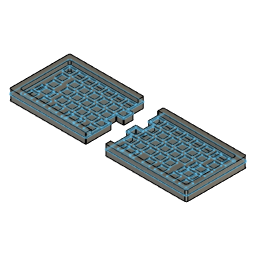
base30_30 (Autodesk Fusion 360 design; units mm, degrees)
Autodesk Fusion 360 part; units mm, degrees
(part 1 of 2)
sketch "kbplate" plane through (0, 0, 0) normal (0, 0, 1) x (1, 0, 0)
  line L0 (231.125, -3.025) -> (231.125, -16.025)
  arc A0 (320.238, -3.025) -> (319.738, -2.525) centre (319.738, -3.025) ccw
  arc A1 (250.175, -16.025) -> (250.675, -16.525) centre (250.675, -16.025) ccw
  line L1 (231.625, -16.525) -> (244.625, -16.525)
  arc A2 (197, -35.575) -> (197.5, -35.075) centre (197, -35.075) ccw
  line L2 (313.738, -17.525) -> (319.738, -17.525)
  line L3 (173.975, -3.025) -> (173.975, -16.025)
  arc A3 (193.025, -16.025) -> (193.525, -16.525) centre (193.525, -16.025) ccw
  arc A4 (212.075, -16.025) -> (212.575, -16.525) centre (212.575, -16.025) ccw
  arc A5 (207.025, -3.025) -> (206.525, -2.525) centre (206.525, -3.025) ccw
  line L4 (250.175, -3.025) -> (250.175, -16.025)
  line L5 (212.575, -16.525) -> (225.575, -16.525)
  line L6 (313.238, -3.025) -> (313.238, -17.025)
  arc A6 (44.6, -35.575) -> (45.1, -35.075) centre (44.6, -35.075) ccw
  arc A7 (297.8, -16.025) -> (298.3, -16.525) centre (298.3, -16.025) ccw
  line L7 (311.8, -16.025) -> (311.8, -3.025)
  arc A8 (250.675, -2.525) -> (250.175, -3.025) centre (250.675, -3.025) ccw
  line L8 (64.15, -35.075) -> (64.15, -22.075)
  arc A9 (197.5, -22.075) -> (197, -21.575) centre (197, -22.075) ccw
  arc A10 (212.575, -2.525) -> (212.075, -3.025) centre (212.575, -3.025) ccw
  line L9 (69.7, -35.575) -> (82.7, -35.575)
  arc A11 (31.1, -35.075) -> (31.6, -35.575) centre (31.6, -35.075) ccw
  arc A12 (183.5, -35.075) -> (184, -35.575) centre (184, -35.075) ccw
  line L10 (320.238, -17.025) -> (320.238, -3.025)
  arc A13 (64.15, -22.075) -> (63.65, -21.575) centre (63.65, -22.075) ccw
  arc A14 (121.3, -22.075) -> (120.8, -21.575) centre (120.8, -22.075) ccw
  line L11 (45.1, -35.075) -> (45.1, -22.075)
  arc A15 (184, -21.575) -> (183.5, -22.075) centre (184, -22.075) ccw
  arc A16 (88.75, -21.575) -> (88.25, -22.075) centre (88.75, -22.075) ccw
  arc A17 (50.15, -35.075) -> (50.65, -35.575) centre (50.65, -35.075) ccw
  arc A18 (101.75, -35.575) -> (102.25, -35.075) centre (101.75, -35.075) ccw
  arc A19 (264.175, -3.025) -> (263.675, -2.525) centre (263.675, -3.025) ccw
  line L12 (206.525, -2.525) -> (193.525, -2.525)
  line L13 (212.075, -3.025) -> (212.075, -16.025)
  arc A20 (69.7, -21.575) -> (69.2, -22.075) centre (69.7, -22.075) ccw
  line L14 (121.3, -35.075) -> (121.3, -22.075)
  line L15 (7.7875, -35.575) -> (20.7875, -35.575)
  arc A21 (313.738, -2.525) -> (313.238, -3.025) centre (313.738, -3.025) ccw
  arc A22 (289.362, -17.025) -> (289.862, -17.525) centre (289.862, -17.025) ccw
  line L16 (283.225, -16.025) -> (283.225, -3.025)
  line L17 (269.225, -3.025) -> (269.225, -16.025)
  line L18 (225.575, -2.525) -> (212.575, -2.525)
  arc A23 (225.575, -16.525) -> (226.075, -16.025) centre (225.575, -16.025) ccw
  arc A24 (226.075, -3.025) -> (225.575, -2.525) centre (225.575, -3.025) ccw
  line L19 (250.675, -16.525) -> (263.675, -16.525)
  arc A25 (263.675, -16.525) -> (264.175, -16.025) centre (263.675, -16.025) ccw
  line L20 (193.025, -3.025) -> (193.025, -16.025)
  line L21 (107.8, -35.575) -> (120.8, -35.575)
  line L22 (120.8, -21.575) -> (107.8, -21.575)
  arc A26 (245.125, -3.025) -> (244.625, -2.525) centre (244.625, -3.025) ccw
  arc A27 (69.2, -35.075) -> (69.7, -35.575) centre (69.7, -35.075) ccw
  line L23 (88.75, -35.575) -> (101.75, -35.575)
  line L24 (184, -35.575) -> (197, -35.575)
  arc A28 (193.525, -2.525) -> (193.025, -3.025) centre (193.525, -3.025) ccw
  arc A29 (21.2875, -22.075) -> (20.7875, -21.575) centre (20.7875, -22.075) ccw
  arc A30 (50.65, -21.575) -> (50.15, -22.075) centre (50.65, -22.075) ccw
  arc A31 (45.1, -22.075) -> (44.6, -21.575) centre (44.6, -22.075) ccw
  line L25 (126.35, -22.075) -> (126.35, -35.075)
  arc A32 (296.362, -3.025) -> (295.862, -2.525) centre (295.862, -3.025) ccw
  line L26 (139.85, -21.575) -> (126.85, -21.575)
  line L27 (7.2875, -22.075) -> (7.2875, -35.075)
  arc A33 (107.8, -21.575) -> (107.3, -22.075) centre (107.8, -22.075) ccw
  line L28 (319.738, -2.525) -> (313.738, -2.525)
  arc A34 (283.225, -3.025) -> (282.725, -2.525) centre (282.725, -3.025) ccw
  line L29 (31.1, -22.075) -> (31.1, -35.075)
  line L30 (69.2, -22.075) -> (69.2, -35.075)
  arc A35 (139.85, -35.575) -> (140.35, -35.075) centre (139.85, -35.075) ccw
  line L31 (50.15, -22.075) -> (50.15, -35.075)
  line L32 (63.65, -21.575) -> (50.65, -21.575)
  line L33 (102.25, -35.075) -> (102.25, -22.075)
  line L34 (50.65, -35.575) -> (63.65, -35.575)
  arc A36 (82.7, -35.575) -> (83.2, -35.075) centre (82.7, -35.075) ccw
  line L35 (88.25, -22.075) -> (88.25, -35.075)
  arc A37 (31.6, -21.575) -> (31.1, -22.075) centre (31.6, -22.075) ccw
  line L36 (107.3, -22.075) -> (107.3, -35.075)
  arc A38 (140.35, -22.075) -> (139.85, -21.575) centre (139.85, -22.075) ccw
  line L37 (140.35, -35.075) -> (140.35, -22.075)
  arc A39 (88.25, -35.075) -> (88.75, -35.575) centre (88.75, -35.075) ccw
  arc A40 (126.85, -21.575) -> (126.35, -22.075) centre (126.85, -22.075) ccw
  line L38 (21.2875, -35.075) -> (21.2875, -22.075)
  line L39 (82.7, -21.575) -> (69.7, -21.575)
  line L40 (44.6, -21.575) -> (31.6, -21.575)
  line L41 (101.75, -21.575) -> (88.75, -21.575)
  arc A41 (20.7875, -35.575) -> (21.2875, -35.075) centre (20.7875, -35.075) ccw
  arc A42 (107.3, -35.075) -> (107.8, -35.575) centre (107.8, -35.075) ccw
  arc A43 (102.25, -22.075) -> (101.75, -21.575) centre (101.75, -22.075) ccw
  line L42 (126.85, -35.575) -> (139.85, -35.575)
  line L43 (31.6, -35.575) -> (44.6, -35.575)
  arc A44 (126.35, -35.075) -> (126.85, -35.575) centre (126.85, -35.075) ccw
  arc A45 (7.2875, -35.075) -> (7.7875, -35.575) centre (7.7875, -35.075) ccw
  line L44 (20.7875, -21.575) -> (7.7875, -21.575)
  arc A46 (63.65, -35.575) -> (64.15, -35.075) centre (63.65, -35.075) ccw
  arc A47 (83.2, -22.075) -> (82.7, -21.575) centre (82.7, -22.075) ccw
  line L45 (83.2, -35.075) -> (83.2, -22.075)
  arc A48 (120.8, -35.575) -> (121.3, -35.075) centre (120.8, -35.075) ccw
  arc A49 (7.7875, -21.575) -> (7.2875, -22.075) centre (7.7875, -22.075) ccw
  line L46 (221.6, -22.075) -> (221.6, -35.075)
  line L47 (316.0625, -21.575) -> (303.0625, -21.575)
  arc A50 (202.55, -35.075) -> (203.05, -35.575) centre (203.05, -35.075) ccw
  line L48 (197.5, -35.075) -> (197.5, -22.075)
  line L49 (303.0625, -35.575) -> (316.0625, -35.575)
  arc A51 (292.25, -35.575) -> (292.75, -35.075) centre (292.25, -35.075) ccw
  line L50 (235.6, -35.075) -> (235.6, -22.075)
  line L51 (222.1, -35.575) -> (235.1, -35.575)
  line L52 (10.1687, -54.625) -> (23.1687, -54.625)
  arc A52 (235.1, -35.575) -> (235.6, -35.075) centre (235.1, -35.075) ccw
  arc A53 (9.6687, -54.125) -> (10.1687, -54.625) centre (10.1687, -54.125) ccw
  arc A54 (303.0625, -21.575) -> (302.5625, -22.075) centre (303.0625, -22.075) ccw
  arc A55 (36.3625, -40.625) -> (35.8625, -41.125) centre (36.3625, -41.125) ccw
  arc A56 (222.1, -21.575) -> (221.6, -22.075) centre (222.1, -22.075) ccw
  line L53 (302.5625, -22.075) -> (302.5625, -35.075)
  line L54 (273.7, -35.075) -> (273.7, -22.075)
  line L55 (36.3625, -54.625) -> (49.3625, -54.625)
  line L56 (23.6687, -54.125) -> (23.6687, -41.125)
  line L57 (292.75, -35.075) -> (292.75, -22.075)
  arc A57 (216.05, -35.575) -> (216.55, -35.075) centre (216.05, -35.075) ccw
  arc A58 (302.5625, -35.075) -> (303.0625, -35.575) centre (303.0625, -35.075) ccw
  arc A59 (254.15, -35.575) -> (254.65, -35.075) centre (254.15, -35.075) ccw
  line L58 (23.1687, -40.625) -> (10.1687, -40.625)
  arc A60 (273.2, -35.575) -> (273.7, -35.075) centre (273.2, -35.075) ccw
  line L59 (235.1, -21.575) -> (222.1, -21.575)
  arc A61 (241.15, -21.575) -> (240.65, -22.075) centre (241.15, -22.075) ccw
  line L60 (273.2, -21.575) -> (260.2, -21.575)
  arc A62 (235.6, -22.075) -> (235.1, -21.575) centre (235.1, -22.075) ccw
  line L61 (292.25, -21.575) -> (279.25, -21.575)
  line L62 (216.55, -35.075) -> (216.55, -22.075)
  line L63 (203.05, -35.575) -> (216.05, -35.575)
  line L64 (241.15, -35.575) -> (254.15, -35.575)
  arc A63 (203.05, -21.575) -> (202.55, -22.075) centre (203.05, -22.075) ccw
  line L65 (202.55, -22.075) -> (202.55, -35.075)
  arc A64 (216.55, -22.075) -> (216.05, -21.575) centre (216.05, -22.075) ccw
  arc A65 (316.0625, -35.575) -> (316.5625, -35.075) centre (316.0625, -35.075) ccw
  line L66 (279.25, -35.575) -> (292.25, -35.575)
  arc A66 (260.2, -21.575) -> (259.7, -22.075) centre (260.2, -22.075) ccw
  line L67 (112.0625, -41.125) -> (112.0625, -54.125)
  arc A67 (169.7125, -40.625) -> (169.2125, -41.125) centre (169.7125, -41.125) ccw
  arc A68 (316.5625, -22.075) -> (316.0625, -21.575) centre (316.0625, -22.075) ccw
  arc A69 (10.1687, -40.625) -> (9.6688, -41.125) centre (10.1687, -41.125) ccw
  arc A70 (49.3625, -54.625) -> (49.8625, -54.125) centre (49.3625, -54.125) ccw
  line L68 (183.5, -22.075) -> (183.5, -35.075)
  arc A71 (183.2125, -41.125) -> (182.7125, -40.625) centre (182.7125, -41.125) ccw
  line L69 (182.7125, -40.625) -> (169.7125, -40.625)
  arc A72 (279.25, -21.575) -> (278.75, -22.075) centre (279.25, -22.075) ccw
  arc A73 (202.2625, -41.125) -> (201.7625, -40.625) centre (201.7625, -41.125) ccw
  arc A74 (54.9125, -54.125) -> (55.4125, -54.625) centre (55.4125, -54.125) ccw
  arc A75 (292.75, -22.075) -> (292.25, -21.575) centre (292.25, -22.075) ccw
  arc A76 (278.75, -35.075) -> (279.25, -35.575) centre (279.25, -35.075) ccw
  arc A77 (273.7, -22.075) -> (273.2, -21.575) centre (273.2, -22.075) ccw
  arc A78 (49.8625, -41.125) -> (49.3625, -40.625) centre (49.3625, -41.125) ccw
  arc A79 (23.6687, -41.125) -> (23.1687, -40.625) centre (23.1687, -41.125) ccw
  arc A80 (207.3125, -54.125) -> (207.8125, -54.625) centre (207.8125, -54.125) ccw
  line L70 (197, -21.575) -> (184, -21.575)
  line L71 (9.6687, -41.125) -> (9.6687, -54.125)
  line L72 (316.5625, -35.075) -> (316.5625, -22.075)
  arc A81 (221.6, -35.075) -> (222.1, -35.575) centre (222.1, -35.075) ccw
  arc A82 (254.65, -22.075) -> (254.15, -21.575) centre (254.15, -22.075) ccw
  line L73 (259.7, -22.075) -> (259.7, -35.075)
  arc A83 (23.1687, -54.625) -> (23.6687, -54.125) centre (23.1687, -54.125) ccw
  line L74 (260.2, -35.575) -> (273.2, -35.575)
  line L75 (254.15, -21.575) -> (241.15, -21.575)
  line L76 (254.65, -35.075) -> (254.65, -22.075)
  line L77 (240.65, -22.075) -> (240.65, -35.075)
  line L78 (216.05, -21.575) -> (203.05, -21.575)
  line L79 (278.75, -22.075) -> (278.75, -35.075)
  arc A84 (259.7, -35.075) -> (260.2, -35.575) centre (260.2, -35.075) ccw
  arc A85 (35.8625, -54.125) -> (36.3625, -54.625) centre (36.3625, -54.125) ccw
  arc A86 (240.65, -35.075) -> (241.15, -35.575) centre (241.15, -35.075) ccw
  line L80 (112.5625, -54.625) -> (125.5625, -54.625)
  arc A87 (188.7625, -40.625) -> (188.2625, -41.125) centre (188.7625, -41.125) ccw
  arc A88 (226.8625, -40.625) -> (226.3625, -41.125) centre (226.8625, -41.125) ccw
  line L81 (183.2125, -54.125) -> (183.2125, -41.125)
  line L82 (226.8625, -54.625) -> (239.8625, -54.625)
  arc A89 (201.7625, -54.625) -> (202.2625, -54.125) centre (201.7625, -54.125) ccw
  arc A90 (182.7125, -54.625) -> (183.2125, -54.125) centre (182.7125, -54.125) ccw
  line L83 (73.9625, -41.125) -> (73.9625, -54.125)
  line L84 (68.9125, -54.125) -> (68.9125, -41.125)
  line L85 (188.7625, -54.625) -> (201.7625, -54.625)
  line L86 (55.4125, -54.625) -> (68.4125, -54.625)
  line L87 (93.5125, -54.625) -> (106.5125, -54.625)
  line L88 (126.0625, -54.125) -> (126.0625, -41.125)
  arc A91 (239.8625, -54.625) -> (240.3625, -54.125) centre (239.8625, -54.125) ccw
  arc A92 (169.2125, -54.125) -> (169.7125, -54.625) centre (169.7125, -54.125) ccw
  line L89 (35.8625, -41.125) -> (35.8625, -54.125)
  line L90 (220.8125, -40.625) -> (207.8125, -40.625)
  arc A93 (112.0625, -54.125) -> (112.5625, -54.625) centre (112.5625, -54.125) ccw
  arc A94 (68.4125, -54.625) -> (68.9125, -54.125) centre (68.4125, -54.125) ccw
  line L91 (107.0125, -54.125) -> (107.0125, -41.125)
  arc A95 (125.5625, -54.625) -> (126.0625, -54.125) centre (125.5625, -54.125) ccw
  arc A96 (74.4625, -40.625) -> (73.9625, -41.125) centre (74.4625, -41.125) ccw
  line L92 (202.2625, -54.125) -> (202.2625, -41.125)
  line L93 (49.3625, -40.625) -> (36.3625, -40.625)
  arc A97 (220.8125, -54.625) -> (221.3125, -54.125) centre (220.8125, -54.125) ccw
  arc A98 (14.4313, -73.175) -> (14.9313, -73.675) centre (14.9313, -73.175) ccw
  line L94 (14.4313, -60.175) -> (14.4313, -73.175)
  arc A99 (12.4932, -74.675) -> (12.9932, -74.175) centre (12.4932, -74.175) ccw
  arc A100 (112.5625, -40.625) -> (112.0625, -41.125) centre (112.5625, -41.125) ccw
  line L95 (125.5625, -40.625) -> (112.5625, -40.625)
  arc A101 (107.0125, -41.125) -> (106.5125, -40.625) centre (106.5125, -41.125) ccw
  line L96 (74.4625, -54.625) -> (87.4625, -54.625)
  arc A102 (93.5125, -40.625) -> (93.0125, -41.125) centre (93.5125, -41.125) ccw
  arc A103 (87.4625, -54.625) -> (87.9625, -54.125) centre (87.4625, -54.125) ccw
  arc A104 (126.0625, -41.125) -> (125.5625, -40.625) centre (125.5625, -41.125) ccw
  line L97 (87.9625, -54.125) -> (87.9625, -41.125)
  arc A105 (73.9625, -54.125) -> (74.4625, -54.625) centre (74.4625, -54.125) ccw
  line L98 (87.4625, -40.625) -> (74.4625, -40.625)
  line L99 (54.9125, -41.125) -> (54.9125, -54.125)
  line L100 (221.3125, -54.125) -> (221.3125, -41.125)
  arc A106 (106.5125, -54.625) -> (107.0125, -54.125) centre (106.5125, -54.125) ccw
  arc A107 (93.0125, -54.125) -> (93.5125, -54.625) centre (93.5125, -54.125) ccw
  arc A108 (240.3625, -41.125) -> (239.8625, -40.625) centre (239.8625, -41.125) ccw
  arc A109 (68.9125, -41.125) -> (68.4125, -40.625) centre (68.4125, -41.125) ccw
  line L101 (106.5125, -40.625) -> (93.5125, -40.625)
  line L102 (68.4125, -40.625) -> (55.4125, -40.625)
  arc A110 (55.4125, -40.625) -> (54.9125, -41.125) centre (55.4125, -41.125) ccw
  line L103 (93.0125, -41.125) -> (93.0125, -54.125)
  line L104 (169.2125, -41.125) -> (169.2125, -54.125)
  line L105 (49.8625, -54.125) -> (49.8625, -41.125)
  arc A111 (188.2625, -54.125) -> (188.7625, -54.625) centre (188.7625, -54.125) ccw
  arc A112 (226.3625, -54.125) -> (226.8625, -54.625) centre (226.8625, -54.125) ccw
  arc A113 (207.8125, -40.625) -> (207.3125, -41.125) centre (207.8125, -41.125) ccw
  line L106 (188.2625, -41.125) -> (188.2625, -54.125)
  arc A114 (87.9625, -41.125) -> (87.4625, -40.625) centre (87.4625, -41.125) ccw
  line L107 (207.3125, -41.125) -> (207.3125, -54.125)
  line L108 (201.7625, -40.625) -> (188.7625, -40.625)
  line L109 (169.7125, -54.625) -> (182.7125, -54.625)
  arc A115 (221.3125, -41.125) -> (220.8125, -40.625) centre (220.8125, -41.125) ccw
  line L110 (207.8125, -54.625) -> (220.8125, -54.625)
  line L111 (278.4625, -54.125) -> (278.4625, -41.125)
  line L112 (245.4125, -41.125) -> (245.4125, -54.125)
  arc A116 (259.4125, -41.125) -> (258.9125, -40.625) centre (258.9125, -41.125) ccw
  line L113 (317.3568, -40.625) -> (311.3568, -40.625)
  arc A117 (311.3567, -40.625) -> (310.8567, -41.125) centre (311.3567, -41.125) ccw
  arc A118 (28.4312, -60.175) -> (27.9312, -59.675) centre (27.9312, -60.175) ccw
  arc A119 (245.4125, -54.125) -> (245.9125, -54.625) centre (245.9125, -54.125) ccw
  arc A120 (309.4187, -41.125) -> (308.9187, -40.625) centre (308.9187, -41.125) ccw
  arc A121 (36.3693, -74.675) -> (36.8693, -74.175) centre (36.3693, -74.175) ccw
  line L114 (317.8567, -55.125) -> (317.8567, -41.125)
  line L115 (5.9932, -60.175) -> (5.9932, -74.175)
  line L116 (309.4187, -54.125) -> (309.4187, -41.125)
  line L117 (293.9808, -55.125) -> (293.9808, -41.125)
  line L118 (258.9125, -40.625) -> (245.9125, -40.625)
  arc A122 (14.9313, -59.675) -> (14.4313, -60.175) centre (14.9313, -60.175) ccw
  arc A123 (293.9808, -41.125) -> (293.4808, -40.625) centre (293.4808, -41.125) ccw
  line L119 (239.8625, -40.625) -> (226.8625, -40.625)
  arc A124 (258.9125, -54.625) -> (259.4125, -54.125) centre (258.9125, -54.125) ccw
  arc A125 (317.8568, -41.125) -> (317.3568, -40.625) centre (317.3568, -41.125) ccw
  arc A126 (6.4933, -59.675) -> (5.9933, -60.175) centre (6.4933, -60.175) ccw
  arc A127 (264.9625, -40.625) -> (264.4625, -41.125) centre (264.9625, -41.125) ccw
  line L120 (28.4313, -73.175) -> (28.4312, -60.175)
  arc A128 (278.4625, -41.125) -> (277.9625, -40.625) centre (277.9625, -41.125) ccw
  arc A129 (317.3568, -55.625) -> (317.8568, -55.125) centre (317.3568, -55.125) ccw
  line L121 (310.8567, -41.125) -> (310.8567, -55.125)
  arc A130 (295.9188, -40.625) -> (295.4188, -41.125) centre (295.9188, -41.125) ccw
  arc A131 (245.9125, -40.625) -> (245.4125, -41.125) centre (245.9125, -41.125) ccw
  arc A132 (295.4188, -54.125) -> (295.9188, -54.625) centre (295.9188, -54.125) ccw
  line L122 (240.3625, -54.125) -> (240.3625, -41.125)
  arc A133 (286.9808, -55.125) -> (287.4808, -55.625) centre (287.4808, -55.125) ccw
  line L123 (27.9312, -59.675) -> (14.9313, -59.675)
  arc A134 (29.8693, -74.175) -> (30.3693, -74.675) centre (30.3693, -74.175) ccw
  line L124 (6.4933, -74.675) -> (12.4932, -74.675)
  arc A135 (27.9312, -73.675) -> (28.4312, -73.175) centre (27.9312, -73.175) ccw
  line L125 (14.9313, -73.675) -> (27.9312, -73.675)
  line L126 (259.4125, -54.125) -> (259.4125, -41.125)
  line L127 (245.9125, -54.625) -> (258.9125, -54.625)
  arc A136 (293.4808, -55.625) -> (293.9808, -55.125) centre (293.4808, -55.125) ccw
  line L128 (36.8693, -74.175) -> (36.8693, -60.175)
  line L129 (211.2875, -59.675) -> (198.2875, -59.675)
  line L130 (12.9932, -74.175) -> (12.9932, -60.175)
  line L131 (311.3567, -55.625) -> (317.3567, -55.625)
  line L132 (192.7375, -73.175) -> (192.7375, -60.175)
  line L133 (12.4932, -59.675) -> (6.4932, -59.675)
  line L134 (308.9187, -40.625) -> (295.9188, -40.625)
  line L135 (293.4808, -40.625) -> (287.4808, -40.625)
  arc A137 (12.9932, -60.175) -> (12.4932, -59.675) centre (12.4932, -60.175) ccw
  arc A138 (36.8693, -60.175) -> (36.3693, -59.675) centre (36.3693, -60.175) ccw
  arc A139 (264.4625, -54.125) -> (264.9625, -54.625) centre (264.9625, -54.125) ccw
  line L136 (295.4187, -41.125) -> (295.4187, -54.125)
  line L137 (295.9188, -54.625) -> (308.9188, -54.625)
  line L138 (287.4808, -55.625) -> (293.4808, -55.625)
  line L139 (286.9808, -41.125) -> (286.9808, -55.125)
  arc A140 (277.9625, -54.625) -> (278.4625, -54.125) centre (277.9625, -54.125) ccw
  line L140 (264.4625, -41.125) -> (264.4625, -54.125)
  arc A141 (287.4808, -40.625) -> (286.9808, -41.125) centre (287.4808, -41.125) ccw
  arc A142 (5.9932, -74.175) -> (6.4933, -74.675) centre (6.4933, -74.175) ccw
  line L141 (277.9625, -40.625) -> (264.9625, -40.625)
  line L142 (30.3693, -74.675) -> (36.3693, -74.675)
  arc A143 (310.8567, -55.125) -> (311.3567, -55.625) centre (311.3567, -55.125) ccw
  arc A144 (308.9187, -54.625) -> (309.4187, -54.125) centre (308.9187, -54.125) ccw
  line L143 (264.9625, -54.625) -> (277.9625, -54.625)
  arc A145 (30.3693, -59.675) -> (29.8693, -60.175) centre (30.3693, -60.175) ccw
  line L144 (226.3625, -41.125) -> (226.3625, -54.125)
  line L145 (178.7375, -60.175) -> (178.7375, -73.175)
  line L146 (197.7875, -60.175) -> (197.7875, -73.175)
  arc A146 (102.5375, -73.175) -> (103.0375, -73.675) centre (103.0375, -73.175) ccw
  arc A147 (211.7875, -60.175) -> (211.2875, -59.675) centre (211.2875, -60.175) ccw
  line L147 (102.5375, -60.175) -> (102.5375, -73.175)
  arc A148 (217.3375, -59.675) -> (216.8375, -60.175) centre (217.3375, -60.175) ccw
  line L148 (29.8693, -60.175) -> (29.8693, -74.175)
  line L149 (45.3875, -60.175) -> (45.3875, -73.175)
  arc A149 (198.2875, -59.675) -> (197.7875, -60.175) centre (198.2875, -60.175) ccw
  line L150 (116.5375, -73.175) -> (116.5375, -60.175)
  arc A150 (192.2375, -73.675) -> (192.7375, -73.175) centre (192.2375, -73.175) ccw
  line L151 (135.5875, -73.175) -> (135.5875, -60.175)
  line L152 (59.3875, -73.175) -> (59.3875, -60.175)
  arc A151 (121.5875, -73.175) -> (122.0875, -73.675) centre (122.0875, -73.175) ccw
  line L153 (78.4375, -73.175) -> (78.4375, -60.175)
  line L154 (179.2375, -73.675) -> (192.2375, -73.675)
  line L155 (211.7875, -73.175) -> (211.7875, -60.175)
  line L156 (103.0375, -73.675) -> (116.0375, -73.675)
  line L157 (83.4875, -60.175) -> (83.4875, -73.175)
  arc A152 (178.7375, -73.175) -> (179.2375, -73.675) centre (179.2375, -73.175) ccw
  arc A153 (97.4875, -60.175) -> (96.9875, -59.675) centre (96.9875, -60.175) ccw
  line L158 (306.5942, -74.675) -> (312.5942, -74.675)
  line L159 (5.4062, -92.725) -> (18.4063, -92.725)
  line L160 (4.9062, -79.225) -> (4.9062, -92.225)
  arc A154 (116.5375, -60.175) -> (116.0375, -59.675) centre (116.0375, -60.175) ccw
  arc A155 (116.0375, -73.675) -> (116.5375, -73.175) centre (116.0375, -73.175) ccw
  arc A156 (64.9375, -59.675) -> (64.4375, -60.175) centre (64.9375, -60.175) ccw
  arc A157 (135.5875, -60.175) -> (135.0875, -59.675) centre (135.0875, -60.175) ccw
  line L161 (45.8875, -73.675) -> (58.8875, -73.675)
  arc A158 (45.8875, -59.675) -> (45.3875, -60.175) centre (45.8875, -60.175) ccw
  line L162 (96.9875, -59.675) -> (83.9875, -59.675)
  arc A159 (64.4375, -73.175) -> (64.9375, -73.675) centre (64.9375, -73.175) ccw
  line L163 (77.9375, -59.675) -> (64.9375, -59.675)
  line L164 (116.0375, -59.675) -> (103.0375, -59.675)
  arc A160 (135.0875, -73.675) -> (135.5875, -73.175) centre (135.0875, -73.175) ccw
  line L165 (83.9875, -73.675) -> (96.9875, -73.675)
  arc A161 (192.7375, -60.175) -> (192.2375, -59.675) centre (192.2375, -60.175) ccw
  arc A162 (230.8375, -60.175) -> (230.3375, -59.675) centre (230.3375, -60.175) ccw
  line L166 (198.2875, -73.675) -> (211.2875, -73.675)
  line L167 (97.4875, -73.175) -> (97.4875, -60.175)
  arc A163 (59.3875, -60.175) -> (58.8875, -59.675) centre (58.8875, -60.175) ccw
  arc A164 (77.9375, -73.675) -> (78.4375, -73.175) centre (77.9375, -73.175) ccw
  arc A165 (83.9875, -59.675) -> (83.4875, -60.175) centre (83.9875, -60.175) ccw
  arc A166 (103.0375, -59.675) -> (102.5375, -60.175) centre (103.0375, -60.175) ccw
  arc A167 (122.0875, -59.675) -> (121.5875, -60.175) centre (122.0875, -60.175) ccw
  line L168 (192.2375, -59.675) -> (179.2375, -59.675)
  arc A168 (211.2875, -73.675) -> (211.7875, -73.175) centre (211.2875, -73.175) ccw
  line L169 (64.4375, -60.175) -> (64.4375, -73.175)
  line L170 (122.0875, -73.675) -> (135.0875, -73.675)
  arc A169 (179.2375, -59.675) -> (178.7375, -60.175) centre (179.2375, -60.175) ccw
  arc A170 (78.4375, -60.175) -> (77.9375, -59.675) centre (77.9375, -60.175) ccw
  arc A171 (197.7875, -73.175) -> (198.2875, -73.675) centre (198.2875, -73.175) ccw
  line L171 (217.3375, -73.675) -> (230.3375, -73.675)
  arc A172 (83.4875, -73.175) -> (83.9875, -73.675) centre (83.9875, -73.175) ccw
  line L172 (135.0875, -59.675) -> (122.0875, -59.675)
  line L173 (64.9375, -73.675) -> (77.9375, -73.675)
  line L174 (58.8875, -59.675) -> (45.8875, -59.675)
  arc A173 (216.8375, -73.175) -> (217.3375, -73.675) centre (217.3375, -73.175) ccw
  arc A174 (45.3875, -73.175) -> (45.8875, -73.675) centre (45.8875, -73.175) ccw
  arc A175 (96.9875, -73.675) -> (97.4875, -73.175) centre (96.9875, -73.175) ccw
  line L175 (121.5875, -60.175) -> (121.5875, -73.175)
  arc A176 (58.8875, -73.675) -> (59.3875, -73.175) centre (58.8875, -73.175) ccw
  arc A177 (230.3375, -73.675) -> (230.8375, -73.175) centre (230.3375, -73.175) ccw
  line L176 (36.3693, -59.675) -> (30.3693, -59.675)
  line L177 (312.5942, -59.675) -> (306.5942, -59.675)
  line L178 (304.6562, -73.175) -> (304.6562, -60.175)
  line L179 (254.9375, -60.175) -> (254.9375, -73.175)
  arc A178 (29.2188, -78.725) -> (28.7188, -79.225) centre (29.2188, -79.225) ccw
  arc A179 (282.7183, -59.675) -> (282.2183, -60.175) centre (282.7183, -60.175) ccw
  line L180 (249.8875, -73.175) -> (249.8875, -60.175)
  line L181 (249.3875, -59.675) -> (236.3875, -59.675)
  line L182 (230.3375, -59.675) -> (217.3375, -59.675)
  arc A180 (288.7183, -74.675) -> (289.2183, -74.175) centre (288.7183, -74.175) ccw
  arc A181 (268.4375, -73.675) -> (268.9375, -73.175) centre (268.4375, -73.175) ccw
  line L183 (282.2183, -60.175) -> (282.2183, -74.175)
  line L184 (291.1562, -73.675) -> (304.1562, -73.675)
  arc A182 (42.7188, -79.225) -> (42.2188, -78.725) centre (42.2188, -79.225) ccw
  line L185 (304.1562, -59.675) -> (291.1562, -59.675)
  arc A183 (268.9375, -60.175) -> (268.4375, -59.675) centre (268.4375, -60.175) ccw
  line L186 (216.8375, -60.175) -> (216.8375, -73.175)
  line L187 (282.7183, -74.675) -> (288.7183, -74.675)
  line L188 (313.0942, -74.175) -> (313.0942, -60.175)
  arc A184 (4.9062, -92.225) -> (5.4062, -92.725) centre (5.4062, -92.225) ccw
  line L189 (289.2183, -74.175) -> (289.2183, -60.175)
  line L190 (268.4375, -59.675) -> (255.4375, -59.675)
  arc A185 (289.2183, -60.175) -> (288.7183, -59.675) centre (288.7183, -60.175) ccw
  line L191 (268.9375, -73.175) -> (268.9375, -60.175)
  line L192 (288.7183, -59.675) -> (282.7183, -59.675)
  arc A186 (249.3875, -73.675) -> (249.8875, -73.175) centre (249.3875, -73.175) ccw
  arc A187 (18.9062, -79.225) -> (18.4062, -78.725) centre (18.4062, -79.225) ccw
  arc A188 (18.4062, -92.725) -> (18.9063, -92.225) centre (18.4062, -92.225) ccw
  arc A189 (28.7188, -92.225) -> (29.2188, -92.725) centre (29.2188, -92.225) ccw
  arc A190 (291.1562, -59.675) -> (290.6562, -60.175) centre (291.1562, -60.175) ccw
  line L193 (29.2188, -92.725) -> (42.2188, -92.725)
  line L194 (42.2188, -78.725) -> (29.2188, -78.725)
  arc A191 (306.0942, -74.175) -> (306.5942, -74.675) centre (306.5942, -74.175) ccw
  line L195 (306.0942, -60.175) -> (306.0942, -74.175)
  line L196 (42.7188, -92.225) -> (42.7188, -79.225)
  line L197 (255.4375, -73.675) -> (268.4375, -73.675)
  arc A192 (290.6562, -73.175) -> (291.1562, -73.675) centre (291.1562, -73.175) ccw
  arc A193 (304.1562, -73.675) -> (304.6562, -73.175) centre (304.1562, -73.175) ccw
  arc A194 (282.2183, -74.175) -> (282.7183, -74.675) centre (282.7183, -74.175) ccw
  line L198 (290.6562, -60.175) -> (290.6562, -73.175)
  arc A195 (304.6562, -60.175) -> (304.1562, -59.675) centre (304.1562, -60.175) ccw
  arc A196 (306.5942, -59.675) -> (306.0942, -60.175) centre (306.5942, -60.175) ccw
  arc A197 (249.8875, -60.175) -> (249.3875, -59.675) centre (249.3875, -60.175) ccw
  line L199 (18.4062, -78.725) -> (5.4062, -78.725)
  arc A198 (42.2188, -92.725) -> (42.7188, -92.225) centre (42.2188, -92.225) ccw
  arc A199 (254.9375, -73.175) -> (255.4375, -73.675) centre (255.4375, -73.175) ccw
  arc A200 (66.5312, -79.225) -> (66.0312, -78.725) centre (66.0312, -79.225) ccw
  arc A201 (312.5942, -74.675) -> (313.0942, -74.175) centre (312.5942, -74.175) ccw
  line L200 (236.3875, -73.675) -> (249.3875, -73.675)
  arc A202 (52.5313, -92.225) -> (53.0313, -92.725) centre (53.0313, -92.225) ccw
  arc A203 (313.0942, -60.175) -> (312.5942, -59.675) centre (312.5942, -60.175) ccw
  line L201 (230.8375, -73.175) -> (230.8375, -60.175)
  arc A204 (66.0312, -92.725) -> (66.5312, -92.225) centre (66.0312, -92.225) ccw
  arc A205 (235.8875, -73.175) -> (236.3875, -73.675) centre (236.3875, -73.175) ccw
  arc A206 (255.4375, -59.675) -> (254.9375, -60.175) centre (255.4375, -60.175) ccw
  line L202 (28.7188, -79.225) -> (28.7188, -92.225)
  line L203 (235.8875, -60.175) -> (235.8875, -73.175)
  line L204 (18.9063, -92.225) -> (18.9063, -79.225)
  arc A207 (5.4062, -78.725) -> (4.9063, -79.225) centre (5.4062, -79.225) ccw
  arc A208 (236.3875, -59.675) -> (235.8875, -60.175) centre (236.3875, -60.175) ccw
  arc A209 (83.9308, -93.725) -> (84.4308, -93.225) centre (83.9308, -93.225) ccw
  line L205 (101.8068, -93.725) -> (107.8068, -93.725)
  line L206 (217.3443, -78.725) -> (211.3442, -78.725)
  arc A210 (247.5063, -79.225) -> (247.0063, -78.725) centre (247.0063, -79.225) ccw
  line L207 (66.0312, -78.725) -> (53.0312, -78.725)
  line L208 (86.3688, -92.725) -> (99.3688, -92.725)
  arc A211 (211.3442, -78.725) -> (210.8442, -79.225) centre (211.3442, -79.225) ccw
  line L209 (53.0313, -92.725) -> (66.0312, -92.725)
  line L210 (66.5312, -92.225) -> (66.5312, -79.225)
  arc A212 (77.4308, -93.225) -> (77.9308, -93.725) centre (77.9308, -93.225) ccw
  line L211 (83.9308, -78.725) -> (77.9308, -78.725)
  arc A213 (186.9683, -93.225) -> (187.4683, -93.725) centre (187.4683, -93.225) ccw
  line L212 (195.9063, -92.725) -> (208.9062, -92.725)
  arc A214 (234.0063, -78.725) -> (233.5063, -79.225) centre (234.0063, -79.225) ccw
  line L213 (209.4062, -92.225) -> (209.4062, -79.225)
  line L214 (186.9683, -79.225) -> (186.9683, -93.225)
  line L215 (234.0063, -92.725) -> (247.0063, -92.725)
  arc A215 (133.2063, -79.225) -> (132.7063, -78.725) centre (132.7063, -79.225) ccw
  line L216 (99.8688, -92.225) -> (99.8688, -79.225)
  line L217 (119.7062, -92.725) -> (132.7063, -92.725)
  arc A216 (195.4063, -92.225) -> (195.9063, -92.725) centre (195.9063, -92.225) ccw
  arc A217 (107.8068, -93.725) -> (108.3068, -93.225) centre (107.8068, -93.225) ccw
  line L218 (119.2063, -79.225) -> (119.2063, -92.225)
  arc A218 (247.0063, -92.725) -> (247.5063, -92.225) centre (247.0063, -92.225) ccw
  arc A219 (210.8442, -93.225) -> (211.3442, -93.725) centre (211.3442, -93.225) ccw
  line L219 (217.8442, -93.225) -> (217.8442, -79.225)
  line L220 (84.4308, -93.225) -> (84.4308, -79.225)
  line L221 (187.4683, -93.725) -> (193.4683, -93.725)
  arc A220 (99.8688, -79.225) -> (99.3688, -78.725) centre (99.3688, -79.225) ccw
  arc A221 (119.7062, -78.725) -> (119.2062, -79.225) centre (119.7062, -79.225) ccw
  arc A222 (84.4308, -79.225) -> (83.9308, -78.725) centre (83.9308, -79.225) ccw
  arc A223 (233.5063, -92.225) -> (234.0063, -92.725) centre (234.0063, -92.225) ccw
  line L222 (77.9308, -93.725) -> (83.9308, -93.725)
  arc A224 (101.3067, -93.225) -> (101.8068, -93.725) centre (101.8068, -93.225) ccw
  arc A225 (101.8068, -78.725) -> (101.3068, -79.225) centre (101.8068, -79.225) ccw
  arc A226 (208.9062, -92.725) -> (209.4062, -92.225) centre (208.9062, -92.225) ccw
  line L223 (193.4683, -78.725) -> (187.4683, -78.725)
  line L224 (211.3442, -93.725) -> (217.3442, -93.725)
  line L225 (208.9062, -78.725) -> (195.9063, -78.725)
  arc A227 (132.7063, -92.725) -> (133.2063, -92.225) centre (132.7063, -92.225) ccw
  arc A228 (119.2062, -92.225) -> (119.7062, -92.725) centre (119.7062, -92.225) ccw
  line L226 (193.9683, -93.225) -> (193.9683, -79.225)
  arc A229 (108.3068, -79.225) -> (107.8068, -78.725) centre (107.8068, -79.225) ccw
  line L227 (195.4063, -79.225) -> (195.4063, -92.225)
  line L228 (101.3067, -79.225) -> (101.3067, -93.225)
  line L229 (85.8688, -79.225) -> (85.8688, -92.225)
  line L230 (133.2063, -92.225) -> (133.2063, -79.225)
  line L231 (107.8068, -78.725) -> (101.8068, -78.725)
  line L232 (210.8442, -79.225) -> (210.8442, -93.225)
  arc A230 (193.9683, -79.225) -> (193.4683, -78.725) centre (193.4683, -79.225) ccw
  arc A231 (209.4062, -79.225) -> (208.9062, -78.725) centre (208.9062, -79.225) ccw
  line L233 (99.3688, -78.725) -> (86.3688, -78.725)
  line L234 (108.3068, -93.225) -> (108.3068, -79.225)
  arc A232 (85.8688, -92.225) -> (86.3688, -92.725) centre (86.3688, -92.225) ccw
  arc A233 (53.0313, -78.725) -> (52.5313, -79.225) centre (53.0313, -79.225) ccw
  arc A234 (195.9063, -78.725) -> (195.4063, -79.225) centre (195.9063, -79.225) ccw
  arc A235 (99.3688, -92.725) -> (99.8688, -92.225) centre (99.3688, -92.225) ccw
  arc A236 (77.9308, -78.725) -> (77.4308, -79.225) centre (77.9308, -79.225) ccw
  line L235 (52.5313, -79.225) -> (52.5313, -92.225)
  arc A237 (187.4683, -78.725) -> (186.9683, -79.225) centre (187.4683, -79.225) ccw
  line L236 (132.7063, -78.725) -> (119.7062, -78.725)
  arc A238 (86.3688, -78.725) -> (85.8688, -79.225) centre (86.3688, -79.225) ccw
  arc A239 (217.8443, -79.225) -> (217.3443, -78.725) centre (217.3443, -79.225) ccw
  arc A240 (217.3443, -93.725) -> (217.8443, -93.225) centre (217.3443, -93.225) ccw
  arc A241 (193.4683, -93.725) -> (193.9683, -93.225) centre (193.4683, -93.225) ccw
  line L237 (77.4308, -79.225) -> (77.4308, -93.225)
  line L238 (174.475, -16.525) -> (187.475, -16.525)
  arc A242 (21.575, -16.025) -> (22.075, -16.525) centre (22.075, -16.025) ccw
  line L239 (294.6313, -78.725) -> (281.6313, -78.725)
  line L240 (3.025, -16.525) -> (16.025, -16.525)
  arc A243 (54.625, -3.025) -> (54.125, -2.525) centre (54.125, -3.025) ccw
  line L241 (60.175, -16.525) -> (73.175, -16.525)
  arc A244 (257.3188, -92.225) -> (257.8188, -92.725) centre (257.8188, -92.225) ccw
  arc A245 (304.9438, -92.225) -> (305.4438, -92.725) centre (305.4438, -92.225) ccw
  line L242 (35.075, -2.525) -> (22.075, -2.525)
  arc A246 (73.175, -16.525) -> (73.675, -16.025) centre (73.175, -16.025) ccw
  line L243 (92.225, -2.525) -> (79.225, -2.525)
  line L244 (305.4438, -92.725) -> (318.4438, -92.725)
  line L245 (130.3254, -2.5361) -> (117.325, -2.525)
  arc A247 (22.075, -2.525) -> (21.575, -3.025) centre (22.075, -3.025) ccw
  line L246 (247.5063, -92.225) -> (247.5063, -79.225)
  line L247 (281.1313, -79.225) -> (281.1313, -92.225)
  arc A248 (111.275, -16.525) -> (111.775, -16.025) centre (111.275, -16.025) ccw
  arc A249 (2.525, -16.025) -> (3.025, -16.525) centre (3.025, -16.025) ccw
  arc A250 (271.3188, -79.225) -> (270.8188, -78.725) centre (270.8188, -79.225) ccw
  line L248 (304.9438, -79.225) -> (304.9437, -92.225)
  line L249 (111.275, -2.525) -> (98.275, -2.525)
  arc A251 (294.6313, -92.725) -> (295.1313, -92.225) centre (294.6313, -92.225) ccw
  arc A252 (60.175, -2.525) -> (59.675, -3.025) centre (60.175, -3.025) ccw
  arc A253 (78.725, -16.025) -> (79.225, -16.525) centre (79.225, -16.025) ccw
  line L250 (40.625, -3.025) -> (40.625, -16.025)
  line L251 (92.725, -16.025) -> (92.725, -3.025)
  line L252 (73.175, -2.525) -> (60.175, -2.525)
  line L253 (16.525, -16.025) -> (16.525, -3.025)
  line L254 (281.6313, -92.725) -> (294.6313, -92.725)
  line L255 (111.775, -16.025) -> (111.775, -3.025)
  arc A254 (41.125, -2.525) -> (40.625, -3.025) centre (41.125, -3.025) ccw
  line L256 (21.575, -3.025) -> (21.575, -16.025)
  arc A255 (318.4438, -92.725) -> (318.9438, -92.225) centre (318.4438, -92.225) ccw
  line L257 (233.5063, -79.225) -> (233.5063, -92.225)
  line L258 (270.8188, -78.725) -> (257.8188, -78.725)
  line L259 (318.9438, -92.225) -> (318.9438, -79.225)
  arc A256 (295.1313, -79.225) -> (294.6313, -78.725) centre (294.6313, -79.225) ccw
  arc A257 (16.525, -3.025) -> (16.025, -2.525) centre (16.025, -3.025) ccw
  arc A258 (318.9438, -79.225) -> (318.4438, -78.725) centre (318.4438, -79.225) ccw
  arc A259 (174.475, -2.525) -> (173.975, -3.025) centre (174.475, -3.025) ccw
  line L260 (295.1313, -92.225) -> (295.1313, -79.225)
  arc A260 (35.575, -3.025) -> (35.075, -2.525) centre (35.075, -3.025) ccw
  arc A261 (92.725, -3.025) -> (92.225, -2.525) centre (92.225, -3.025) ccw
  line L261 (257.3188, -79.225) -> (257.3188, -92.225)
  arc A262 (305.4438, -78.725) -> (304.9438, -79.225) centre (305.4438, -79.225) ccw
  line L262 (318.4438, -78.725) -> (305.4438, -78.725)
  arc A263 (116.825, -16.025) -> (117.325, -16.525) centre (117.325, -16.025) ccw
  line L263 (271.3188, -92.225) -> (271.3188, -79.225)
  arc A264 (111.775, -3.025) -> (111.275, -2.525) centre (111.275, -3.025) ccw
  arc A265 (257.8188, -78.725) -> (257.3188, -79.225) centre (257.8188, -79.225) ccw
  line L264 (41.125, -16.525) -> (54.125, -16.525)
  arc A266 (281.1313, -92.225) -> (281.6313, -92.725) centre (281.6313, -92.225) ccw
  arc A267 (40.625, -16.025) -> (41.125, -16.525) centre (41.125, -16.025) ccw
  arc A268 (35.075, -16.525) -> (35.575, -16.025) centre (35.075, -16.025) ccw
  line L265 (247.0063, -78.725) -> (234.0063, -78.725)
  arc A269 (92.225, -16.525) -> (92.725, -16.025) centre (92.225, -16.025) ccw
  line L266 (257.8188, -92.725) -> (270.8188, -92.725)
  arc A270 (54.125, -16.525) -> (54.625, -16.025) centre (54.125, -16.025) ccw
  arc A271 (117.325, -2.525) -> (116.825, -3.025) centre (117.325, -3.025) ccw
  arc A272 (281.6313, -78.725) -> (281.1313, -79.225) centre (281.6313, -79.225) ccw
  line L267 (16.025, -2.525) -> (3.025, -2.525)
  line L268 (35.575, -16.025) -> (35.575, -3.025)
  arc A273 (270.8188, -92.725) -> (271.3188, -92.225) centre (270.8188, -92.225) ccw
  line L269 (117.325, -16.525) -> (130.3253, -16.518)
  line L270 (264.175, -16.025) -> (264.175, -3.025)
  arc A274 (59.675, -16.025) -> (60.175, -16.525) centre (60.175, -16.025) ccw
  line L271 (311.3, -2.525) -> (298.3, -2.525)
  line L272 (289.362, -3.025) -> (289.362, -17.025)
  arc A275 (3.025, -2.525) -> (2.525, -3.025) centre (3.025, -3.025) ccw
  arc A276 (231.125, -16.025) -> (231.625, -16.525) centre (231.625, -16.025) ccw
  line L273 (78.725, -3.025) -> (78.725, -16.025)
  arc A277 (173.975, -16.025) -> (174.475, -16.525) centre (174.475, -16.025) ccw
  arc A278 (206.525, -16.525) -> (207.025, -16.025) centre (206.525, -16.025) ccw
  arc A279 (295.862, -17.525) -> (296.362, -17.025) centre (295.862, -17.025) ccw
  line L274 (269.725, -16.525) -> (282.725, -16.525)
  arc A280 (269.725, -2.525) -> (269.225, -3.025) centre (269.725, -3.025) ccw
  arc A281 (289.862, -2.525) -> (289.362, -3.025) centre (289.862, -3.025) ccw
  line L275 (289.862, -17.525) -> (295.862, -17.525)
  line L276 (297.8, -3.025) -> (297.8, -16.025)
  line L277 (98.275, -16.525) -> (111.275, -16.525)
  line L278 (54.625, -16.025) -> (54.625, -3.025)
  line L279 (187.975, -16.025) -> (187.975, -3.025)
  line L280 (226.075, -16.025) -> (226.075, -3.025)
  line L281 (244.625, -2.525) -> (231.625, -2.525)
  line L282 (97.775, -3.025) -> (97.775, -16.025)
  arc A282 (282.725, -16.525) -> (283.225, -16.025) centre (282.725, -16.025) ccw
  line L283 (2.525, -3.025) -> (2.525, -16.025)
  line L284 (207.025, -16.025) -> (207.025, -3.025)
  line L285 (263.675, -2.525) -> (250.675, -2.525)
  line L286 (296.362, -17.025) -> (296.362, -3.025)
  line L287 (193.525, -16.525) -> (206.525, -16.525)
  line L288 (282.725, -2.525) -> (269.725, -2.525)
  line L289 (298.3, -16.525) -> (311.3, -16.525)
  arc A283 (313.238, -17.025) -> (313.738, -17.525) centre (313.738, -17.025) ccw
  arc A284 (97.775, -16.025) -> (98.275, -16.525) centre (98.275, -16.025) ccw
  arc A285 (187.475, -16.525) -> (187.975, -16.025) centre (187.475, -16.025) ccw
  arc A286 (16.025, -16.525) -> (16.525, -16.025) centre (16.025, -16.025) ccw
  line L290 (59.675, -3.025) -> (59.675, -16.025)
  arc A287 (79.225, -2.525) -> (78.725, -3.025) centre (79.225, -3.025) ccw
  arc A288 (244.625, -16.525) -> (245.125, -16.025) centre (244.625, -16.025) ccw
  arc A289 (319.738, -17.525) -> (320.238, -17.025) centre (319.738, -17.025) ccw
  arc A290 (311.8, -3.025) -> (311.3, -2.525) centre (311.3, -3.025) ccw
  arc A291 (231.625, -2.525) -> (231.125, -3.025) centre (231.625, -3.025) ccw
  line L291 (79.225, -16.525) -> (92.225, -16.525)
  line L292 (73.675, -16.025) -> (73.675, -3.025)
  line L293 (295.862, -2.525) -> (289.862, -2.525)
  arc A292 (98.275, -2.525) -> (97.775, -3.025) centre (98.275, -3.025) ccw
  arc A293 (73.675, -3.025) -> (73.175, -2.525) centre (73.175, -3.025) ccw
  line L294 (245.125, -16.025) -> (245.125, -3.025)
  arc A294 (187.975, -3.025) -> (187.475, -2.525) centre (187.475, -3.025) ccw
  line L295 (116.825, -3.025) -> (116.825, -16.025)
  line L296 (54.125, -2.525) -> (41.125, -2.525)
  arc A295 (311.3, -16.525) -> (311.8, -16.025) centre (311.3, -16.025) ccw
  line L297 (187.475, -2.525) -> (174.475, -2.525)
  line L298 (22.075, -16.525) -> (35.075, -16.525)
  arc A296 (298.3, -2.525) -> (297.8, -3.025) centre (298.3, -3.025) ccw
  arc A297 (269.225, -16.025) -> (269.725, -16.525) centre (269.725, -16.025) ccw
  line L299 (132.35, 0.475) -> (2.525, 0.475)
  line L300 (-0.475, -2.525) -> (-0.475, -93.725)
  line L301 (2.525, -96.725) -> (137.1125, -96.725)
  line L302 (323.238, -93.725) -> (323.238, -2.525)
  line L303 (142.875, -37.1) -> (142.875, -20.05)
  line L304 (141.875, -19.05) -> (134.35, -19.05)
  line L305 (129.5875, -38.1) -> (141.875, -38.1)
  line L306 (128.5875, -56.15) -> (128.5875, -39.1)
  line L307 (137.1125, -57.15) -> (129.5875, -57.15)
  line L308 (138.1125, -105.725) -> (138.1125, -58.15)
  line L309 (177.2125, -96.725) -> (320.238, -96.725)
  line L310 (171.45, 9.475) -> (171.45, -18.05)
  line L311 (320.238, 0.475) -> (172.45, 0.475)
  line L312 (172.45, -19.05) -> (179.975, -19.05)
  line L313 (180.975, -20.05) -> (180.975, -37.1)
  line L314 (179.975, -38.1) -> (167.6875, -38.1)
  line L315 (166.6875, -39.1) -> (166.6875, -56.15)
  line L316 (167.6875, -57.15) -> (175.2125, -57.15)
  line L317 (176.2125, -58.15) -> (176.2125, -105.725)
  arc A298 (2.525, 0.475) -> (-0.475, -2.525) centre (2.525, -2.525) ccw
  arc A299 (-0.475, -93.725) -> (2.525, -96.725) centre (2.525, -93.725) ccw
  arc A300 (137.1125, -96.725) -> (138.1125, -95.725) centre (137.1125, -95.725) ccw
  arc A301 (138.1125, -58.15) -> (137.1125, -57.15) centre (137.1125, -58.15) ccw
  arc A302 (128.5875, -56.15) -> (129.5875, -57.15) centre (129.5875, -56.15) ccw
  arc A303 (129.5875, -38.1) -> (128.5875, -39.1) centre (129.5875, -39.1) ccw
  arc A304 (141.875, -38.1) -> (142.875, -37.1) centre (141.875, -37.1) ccw
  arc A305 (142.875, -20.05) -> (141.875, -19.05) centre (141.875, -20.05) ccw
  arc A306 (171.45, -18.05) -> (172.45, -19.05) centre (172.45, -18.05) ccw
  arc A307 (180.975, -20.05) -> (179.975, -19.05) centre (179.975, -20.05) ccw
  arc A308 (179.975, -38.1) -> (180.975, -37.1) centre (179.975, -37.1) ccw
  arc A309 (167.6875, -38.1) -> (166.6875, -39.1) centre (167.6875, -39.1) ccw
  arc A310 (166.6875, -56.15) -> (167.6875, -57.15) centre (167.6875, -56.15) ccw
  arc A311 (176.2125, -58.15) -> (175.2125, -57.15) centre (175.2125, -58.15) ccw
  arc A312 (176.2125, -95.725) -> (177.2125, -96.725) centre (177.2125, -95.725) ccw
  arc A313 (320.238, -96.725) -> (323.238, -93.725) centre (320.238, -93.725) ccw
  arc A314 (172.45, 0.475) -> (171.45, -0.525) centre (172.45, -0.525) ccw
  arc A315 (323.238, -2.525) -> (320.238, 0.475) centre (320.238, -2.525) ccw
  line L318 (-7.475, -106.725) -> (137.1125, -106.725)
  line L319 (-10.475, 7.475) -> (-10.475, -103.725)
  line L320 (132.35, 10.475) -> (-7.475, 10.475)
  line L321 (330.238, 10.475) -> (172.45, 10.475)
  line L322 (333.238, -103.725) -> (333.238, 7.475)
  line L323 (177.2125, -106.725) -> (330.238, -106.725)
  arc A316 (-7.475, 10.475) -> (-10.475, 7.475) centre (-7.475, 7.475) ccw
  arc A317 (-10.475, -103.725) -> (-7.475, -106.725) centre (-7.475, -103.725) ccw
  arc A318 (137.1125, -106.725) -> (138.1125, -105.725) centre (137.1125, -105.725) ccw
  arc A319 (176.2125, -105.725) -> (177.2125, -106.725) centre (177.2125, -105.725) ccw
  arc A320 (172.45, 10.475) -> (171.45, 9.475) centre (172.45, 9.475) ccw
  arc A321 (333.238, 7.475) -> (330.238, 10.475) centre (330.238, 7.475) ccw
  arc A322 (330.238, -106.725) -> (333.238, -103.725) centre (330.238, -103.725) ccw
  line L324 (130.825, -3.0361) -> (130.825, -16.018)
  arc A323 (130.825, -3.0361) -> (130.3254, -2.5361) centre (130.325, -3.0361) ccw
  arc A324 (130.3253, -16.518) -> (130.825, -16.018) centre (130.325, -16.018) ccw
  line L325 (133.35, 9.475) -> (133.35, -18.05)
  arc A325 (133.35, -0.525) -> (132.35, 0.475) centre (132.35, -0.525) ccw
  arc A326 (133.35, -18.05) -> (134.35, -19.05) centre (134.35, -18.05) ccw
  arc A327 (133.35, 9.475) -> (132.35, 10.475) centre (132.35, 9.475) ccw
  line L326 (136.1125, -105.725) -> (136.1125, -60.15)
  line L327 (135.1125, -59.15) -> (127.5875, -59.15)
  line L328 (126.5875, -58.15) -> (126.5875, -37.1)
  line L329 (127.5875, -36.1) -> (139.875, -36.1)
  line L330 (140.875, -35.1) -> (140.875, -22.05)
  line L331 (139.875, -21.05) -> (132.35, -21.05)
  line L332 (131.35, 9.475) -> (131.35, -20.05)
  arc A328 (136.1125, -60.15) -> (135.1125, -59.15) centre (135.1125, -60.15) ccw
  arc A329 (126.5875, -58.15) -> (127.5875, -59.15) centre (127.5875, -58.15) ccw
  arc A330 (127.5875, -36.1) -> (126.5875, -37.1) centre (127.5875, -37.1) ccw
  arc A331 (139.875, -36.1) -> (140.875, -35.1) centre (139.875, -35.1) ccw
  arc A332 (140.875, -22.05) -> (139.875, -21.05) centre (139.875, -22.05) ccw
  arc A333 (131.35, -20.05) -> (132.35, -21.05) centre (132.35, -20.05) ccw
  line L333 (178.2125, -56.15) -> (178.2125, -105.725)
  line L334 (169.6875, -55.15) -> (177.2125, -55.15)
  line L335 (168.6875, -41.1) -> (168.6875, -54.15)
  line L336 (181.975, -40.1) -> (169.6875, -40.1)
  line L337 (182.975, -18.05) -> (182.975, -39.1)
  line L338 (174.45, -17.05) -> (181.975, -17.05)
  line L339 (173.45, 9.475) -> (173.45, -16.05)
  arc A334 (173.45, -16.05) -> (174.45, -17.05) centre (174.45, -16.05) ccw
  arc A335 (182.975, -18.05) -> (181.975, -17.05) centre (181.975, -18.05) ccw
  arc A336 (181.975, -40.1) -> (182.975, -39.1) centre (181.975, -39.1) ccw
  arc A337 (169.6875, -40.1) -> (168.6875, -41.1) centre (169.6875, -41.1) ccw
  arc A338 (168.6875, -54.15) -> (169.6875, -55.15) centre (169.6875, -54.15) ccw
  arc A339 (178.2125, -56.15) -> (177.2125, -55.15) centre (177.2125, -56.15) ccw
  dimension "d23" = 3
  dimension "d24" = 3
  dimension "d26" = 1
  dimension "d27" = 1
  dimension "d28" = 1
  dimension "d29" = 1
  dimension "d30" = 1
  dimension "d31" = 1
  dimension "d35" = 1
  dimension "d36" = 1
  dimension "d37" = 1
  dimension "d39" = 1
  dimension "d40" = 1
  dimension "d41" = 3
  dimension "d42" = 1
  dimension "d43" = 3
  dimension "d50" = 3
  dimension "d51" = 3
  dimension "d53" = 1
  dimension "d54" = 1
  dimension "d55" = 1
  dimension "d56" = 3
  dimension "d57" = 3
  dimension "d87" = 0.5
  dimension "d88" = 0.5
  dimension "d90" = 1
  dimension "d91" = 1
  dimension "d92" = 1
  dimension "d100" = 1
  dimension "d101" = 1
  dimension "d102" = 1
  dimension "d103" = 1
  dimension "d104" = 1
  dimension "d105" = 1
  dimension "d113" = 1
  dimension "d114" = 1
  dimension "d115" = 1
  dimension "d116" = 1
  dimension "d117" = 1
  dimension "d118" = 1
  constraint parallel L267 L299
  constraint parallel L283 L300
  constraint tangent L299 A298
  constraint tangent L300 A298
  constraint parallel L222 L301
  constraint tangent L300 A299
  constraint tangent L301 A299
  constraint parallel L151 L308
  constraint tangent L301 A300
  constraint tangent L308 A300
  constraint parallel L172 L307
  constraint tangent L308 A301
  constraint tangent L307 A301
  constraint parallel L88 L306
  constraint tangent L307 A302
  constraint tangent L306 A302
  constraint parallel L42 L305
  constraint tangent L306 A303
  constraint tangent L305 A303
  constraint parallel L37 L303
  constraint tangent L303 A304
  constraint tangent L305 A304
  constraint tangent L303 A305
  constraint tangent L304 A305
  constraint tangent L310 A306
  constraint tangent L312 A306
  constraint tangent L312 A307
  constraint tangent L313 A307
  constraint tangent L313 A308
  constraint tangent L314 A308
  constraint tangent L314 A309
  constraint tangent L315 A309
  constraint tangent L315 A310
  constraint tangent L316 A310
  constraint tangent L316 A311
  constraint tangent L317 A311
  constraint tangent L317 A312
  constraint tangent L309 A312
  constraint tangent L309 A313
  constraint tangent L302 A313
  constraint tangent L310 A314
  constraint tangent L311 A314
  constraint tangent L311 A315
  constraint tangent L302 A315
  constraint tangent L320 A316
  constraint tangent L319 A316
  constraint tangent L319 A317
  constraint tangent L318 A317
  constraint coincident L308 A300.end
  constraint tangent L318 A318
  constraint tangent L308 A318
  constraint coincident L317 A312.start
  constraint tangent L317 A319
  constraint tangent L323 A319
  constraint coincident L310 A314.end
  constraint tangent L310 A320
  constraint tangent L321 A320
  constraint tangent L321 A321
  constraint tangent L322 A321
  constraint tangent L322 A322
  constraint tangent L323 A322
  constraint tangent L245 A323
  constraint tangent L324 A323
  constraint tangent L269 A324
  constraint tangent L324 A324
  constraint tangent L299 A325
  constraint tangent L325 A325
  constraint tangent L325 A326
  constraint tangent L304 A326
  constraint coincident L325 A325.start
  constraint tangent L320 A327
  constraint tangent L325 A327
  constraint tangent L326 A328
  constraint tangent L327 A328
  constraint tangent L327 A329
  constraint tangent L328 A329
  constraint tangent L329 A330
  constraint tangent L328 A330
  constraint tangent L329 A331
  constraint tangent L330 A331
  constraint tangent L331 A332
  constraint tangent L330 A332
  constraint tangent L331 A333
  constraint tangent L332 A333
  constraint tangent L339 A334
  constraint tangent L338 A334
  constraint tangent L337 A335
  constraint tangent L338 A335
  constraint tangent L336 A336
  constraint tangent L337 A336
  constraint tangent L335 A337
  constraint tangent L336 A337
  constraint tangent L335 A338
  constraint tangent L334 A338
  constraint tangent L333 A339
  constraint tangent L334 A339
  measures "d23" radius of A298
  measures "d24" radius of A299
  measures "d26" radius of A300
  measures "d27" radius of A301
  measures "d28" radius of A302
  measures "d29" radius of A303
  measures "d30" radius of A304
  measures "d31" radius of A305
  measures "d35" radius of A307
  measures "d36" radius of A308
  measures "d37" radius of A309
  measures "d39" radius of A311
  measures "d40" radius of A312
  measures "d41" radius of A313
  measures "d42" radius of A314
  measures "d43" radius of A315